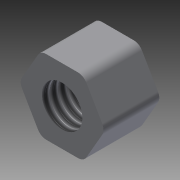
# Autodesk Inventor part: CNC-1.1v-B-1-( nut )
Saved by Autodesk Inventor 2015 (Build 190159000, 159)
## iProperties
Created: 2015-07-11
Part Number: CNC-1.1v-B-1-( nut )
Material: Generic
Document SubType Name: Modeling
Designer: Bangladesh
Density: 1 g/cm^3
Appearance: Default
Author: Bangladesh
Autodesk Inventor part; units mm, degrees
ref_plane "YZ Plane" through (0, 0, 0) normal (1, 0, 0) x (0, 1, 0)
ref_plane "XZ Plane" through (0, 0, 0) normal (0, 1, 0) x (-1, 0, 0)
ref_plane "XY Plane" through (0, 0, 0) normal (0, 0, 1) x (1, 0, 0)
sketch "Sketch1" plane through (0, 0, 0) normal (0, 0, 1) x (1, 0, 0)
  circle A0 centre (0, 0) radius 7.15
  line L0 (-7.15, 0) -> (-3.575, 6.1921)
  line L1 (-3.575, 6.1921) -> (3.575, 6.1921)
  line L2 (3.575, 6.1921) -> (7.15, 0)
  line L3 (7.15, 0) -> (3.575, -6.1921)
  line L4 (3.575, -6.1921) -> (-3.575, -6.1921)
  line L5 (-3.575, -6.1921) -> (-7.15, 0)
  dimension "d0" = 14.3
  constraints: 12 end point, 2 coincident, 1 horizontal alignment, 15 other
extrude "Extrusion1" add sketch "Sketch1" along normal mid plane 9.3 contours L3 L4 L5 L0 L1 L2
sketch "Sketch2" plane through (0, 0, 4.65) normal (0, 0, 1) x (1, 0, 0)
  point P0 (0, 0)
hole "Hole1" at (0, 0, 4.65) direction (0, 0, -1) diameter 6.75 end through all
thread "Thread1" size "5/16-18 UNC" class "2B" standard "ANSI Unified Screw Threads" full length
fillet "Fillet1" radius 1.5875 6 edges at (-3.575, -6.1921, 0) (-7.15, 0, 0) (-3.575, 6.1921, 0) (3.575, 6.1921, 0) (7.15, 0, 0) (3.575, -6.1921, 0)
body "Solid1"
